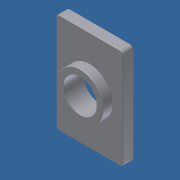
# Autodesk Inventor part: SM-H11
Saved by Autodesk Inventor 2012 SP1 (Build 160190100, 190)
## iProperties
Created: 2012-01-26
Part Number: SM-H11
Material: Steel, Mild
Document SubType Name: Modeling
Designer: ERF
Mass: 1.83016 g
Surface Area: 4.11237 cm^2
Volume: 0.232845 cm^3
Density: 7.86 g/cm^3
Description: pre-assembly insertion nuts (misumi)
Stock Number: HNKK5
Vendor: Misumi
Project: Shapeoko
Author: ERF
Title: Insertion Nut
Autodesk Inventor part; units mm, degrees
ref_plane "YZ Plane" through (0, 0, 0) normal (1, 0, 0) x (0, 1, 0)
ref_plane "XZ Plane" through (0, 0, 0) normal (0, 1, 0) x (-1, 0, 0)
ref_plane "XY Plane" through (0, 0, 0) normal (0, 0, 1) x (1, 0, 0)
sketch "Sketch1" plane through (0, 0, 0) normal (0, 0, 1) x (1, 0, 0)
  line L0 (4.3682, 17.1217) -> (14.3682, 17.1217)
  line L1 (14.3682, 17.1217) -> (14.3682, 2.1217)
  line L2 (14.3682, 2.1217) -> (4.3682, 2.1217)
  line L3 (4.3682, 2.1217) -> (4.3682, 17.1217)
  dimension "d0" = 10
  dimension "d1" = 15
  constraints: 8 end point, 2 parallel, 1 horizontal, 1 perpendicular
  measures "d0" distance of L0.start L0.end
  measures "d1" distance of L0.end L1.end
extrude "Extrusion1" add sketch "Sketch1" along normal blind 1.6
sketch "Sketch2" plane through (0, 0, 1.6) normal (0, 0, 1) x (1, 0, 0)
  line L0 (4.3682, 17.1217) -> (14.3682, 17.1217) projected
  line L1 (4.3682, 2.1217) -> (4.3682, 17.1217) projected
  circle A0 centre (9.3682, 9.6217) radius 3.45
  dimension "d4" = 6.9
  dimension "d5" = 5
  dimension "d6" = 7.5
  constraints: 1 centre point
  measures "d4" diameter of A0
  measures "d5" distance from line of L1 A0.centre
  measures "d6" distance from line of L0 A0.centre
extrude "Extrusion2" add sketch "Sketch2" along normal blind 1.4
sketch "Sketch3" plane through (9.3682, 9.6217, 3) normal (0, 0, 1) x (1, 0, 0)
  circle A0 centre (0, 0) radius 3.45 projected
  circle A1 centre (0, 0) radius 2.5
  dimension "d9" = 5
  constraints: 1 centre point, 1 coincident
  measures "d9" diameter of A1
extrude "Extrusion3" cut sketch "Sketch3" against normal through all contours A1
fillet "Fillet1" radius 0.5 4 edges at (14.3682, 17.1217, 0.8) (14.3682, 2.1217, 0.8) (4.3682, 2.1217, 0.8) (4.3682, 17.1217, 0.8)
fillet "Fillet2" radius 0.1 17 edges at (5.9182, 9.6217, 3) (14.3682, 9.6217, 1.6) (14.2217, 2.2681, 1.6) (9.3682, 2.1217, 1.6) (4.5146, 2.2681, 1.6) (4.3682, 9.6217, 1.6) (4.5146, 16.9752, 1.6) (9.3682, 17.1217, 1.6) (14.2217, 16.9752, 1.6) (14.3682, 9.6217, 0) (14.2217, 2.2681, 0) (9.3682, 2.1217, 0) (4.5146, 2.2681, 0) (4.3682, 9.6217, 0) (4.5146, 16.9752, 0) (9.3682, 17.1217, 0) (14.2217, 16.9752, 0)
body "Solid1"
